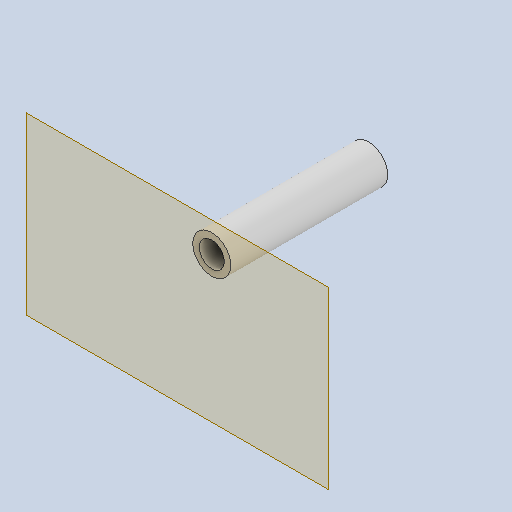
# Autodesk Inventor part: pin_V3
Saved by Autodesk Inventor 2023 (Build 270158000, 158)
## iProperties
Created: 2022-11-25
Part Number: pin_V3
Material: Generic
Document SubType Name: Modeling
Designer: shrey
Density: 1 g/cm^3
Appearance: Default
Author: shrey
Autodesk Inventor part; units mm, degrees
ref_plane "YZ Plane" through (0, 0, 0) normal (1, 0, 0) x (0, 1, 0)
ref_plane "XZ Plane" through (0, 0, 0) normal (0, 1, 0) x (-1, 0, 0)
ref_plane "Work Plane1" through (-60.9685, -13.6118, 33.2922) normal (0, 0, 1) x (1, 0, 0)
sketch "Sketch1" plane through (-60.9685, -13.6118, 33.2922) normal (0, 0, 1) x (1, 0, 0)
  circle A0 centre (10.5928, 20.0161) radius 6.16 construction
  circle A1 centre (10.5928, 20.0161) radius 5.86
  circle A2 centre (10.5928, 20.0161) radius 3.86
  point P0 (60.9685, 13.6118)
  dimension "d0" = 0.3
  dimension "d1" = 2
  constraints: 2 centre point
  measures "d0" radial gap between concentric circles of A0 A1
  measures "d1" radial gap between concentric circles of A1 A2
ref_plane "Work Plane2" through (-103.5613, -36.0957, -15.2678) normal (0, 0, -1) x (0, 1, 0)
extrude "Extrusion1" add sketch "Sketch1" against normal up to surface (48.56 mm away)
body "Solid1"
